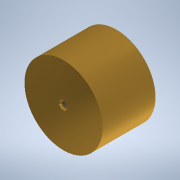
# Autodesk Inventor part: CounterWeights_Brass
Saved by Autodesk Inventor 2021.4 (Build 254397000, 397)
## iProperties
Created: 2022-07-01
Part Number: CounterWeights_Brass
Material: Brass, Soft Yellow
Document SubType Name: Modeling
Designer: alexw
Density: 8.47 g/cm^3
Appearance: Brass - Satin
Mass: 287.838 g
Surface Area: 59.9808 cm^2
Volume: 33.9833 cm^3
Author: alexw
Autodesk Inventor part; units mm, degrees
ref_plane "YZ Plane" through (0, 0, 0) normal (1, 0, 0) x (0, 1, 0)
ref_plane "XZ Plane" through (0, 0, 0) normal (0, 1, 0) x (-1, 0, 0)
ref_plane "XY Plane" through (0, 0, 0) normal (0, 0, 1) x (1, 0, 0)
sketch "Sketch1" plane through (0, 0, 0) normal (0, 0, 1) x (1, 0, 0)
  circle A0 centre (0, 0) radius 20
  dimension "d0" = 40
  constraints: 1 centre point, 1 coincident
  measures "d0" diameter of A0
extrude "Extrusion1" add sketch "Sketch1" along normal blind 27.1
sketch "Sketch2" plane through (0, 0, 27.1) normal (0, 0, 1) x (1, 0, 0)
  point P0 (0, 0)
  point P1 (0, 0)
  constraints: 1 coincident
hole "Hole1" at (0, 0, 27.1) direction (0, 0, -1) diameter 3.242 depth 8 tip angle 118 thread size "M4x0.7" class "6H" standard "ISO Metric profile"
chamfer "Chamfer1" distance 0.7 angle 45 1 edges at (0, 1.621, 27.1)
body "Solid1"
